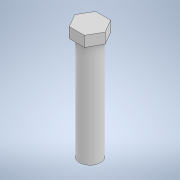
# Autodesk Inventor part: trail 14
Saved by Autodesk Inventor 2020.2 (Build 242310000, 310)
## iProperties
Created: 2020-02-27
Part Number: trail 14
Material: Generic
Document SubType Name: Modeling
Designer: lenovo
Density: 1 g/cm^3
Appearance: Default
Author: lenovo
Autodesk Inventor part; units mm, degrees
ref_plane "YZ Plane" through (0, 0, 0) normal (1, 0, 0) x (0, 1, 0)
ref_plane "XZ Plane" through (0, 0, 0) normal (0, 1, 0) x (-1, 0, 0)
ref_plane "XY Plane" through (0, 0, 0) normal (0, 0, 1) x (1, 0, 0)
sketch "Sketch1" plane through (0, 0, 0) normal (0, 1, 0) x (-1, 0, 0)
  circle A0 centre (0, 0) radius 1
  dimension "d0" = 2
  constraints: 1 centre point, 1 coincident
  measures "d0" diameter of A0
extrude "Extrusion1" add sketch "Sketch1" along normal blind 10
sketch "Sketch2" plane through (0, 10, 0) normal (0, 1, 0) x (1, 0, 0)
  line L0 (-0.7217, -1.25) -> (-1.4434, 0)
  line L1 (-1.4434, 0) -> (-0.7217, 1.25)
  line L2 (-0.7217, 1.25) -> (0.7217, 1.25)
  line L3 (0.7217, 1.25) -> (1.4434, 0)
  line L4 (1.4434, 0) -> (0.7217, -1.25)
  line L5 (0.7217, -1.25) -> (-0.7217, -1.25)
  point P0 (0, 0)
  point P1 (0, 0)
  dimension "d3" = 2.5
  constraints: 12 end point, 1 coincident, 13 other
  measures "d3" distance between parallel lines of L2 L5
extrude "Extrusion2" add sketch "Sketch2" along normal blind 1
body "Solid1"
